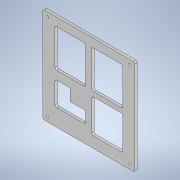
# Autodesk Inventor part: AssemblyPlate
Saved by Autodesk Inventor 2021 (Build 250183000, 183)
## iProperties
Created: 2020-11-06
Part Number: AssemblyPlate
Material: Generic
Document SubType Name: Modeling
Designer: lgnds
Density: 1 g/cm^3
Appearance: Default
Author: lgnds
Autodesk Inventor part; units mm, degrees
ref_plane "YZ Plane" through (0, 0, 0) normal (1, 0, 0) x (0, 1, 0)
ref_plane "XZ Plane" through (0, 0, 0) normal (0, 1, 0) x (-1, 0, 0)
ref_plane "XY Plane" through (0, 0, 0) normal (0, 0, 1) x (1, 0, 0)
sketch "Sketch1" plane through (0, 0, 0) normal (0, 0, 1) x (1, 0, 0)
  line L0 (-56, -58) -> (56, -58)
  line L1 (56, -58) -> (56, 58)
  line L2 (56, 58) -> (-56, 58)
  line L3 (-56, 58) -> (-56, -58)
  line L4 (-56, -58) -> (56, 58) construction
  line L5 (56, -58) -> (-56, 58) construction
  point P0 (0, 0)
  dimension "d0" = 116
  dimension "d1" = 112
  constraints: 12 end point, 2 midpoint, 2 parallel, 1 horizontal, 1 perpendicular
  measures "d0" distance between parallel lines of L0 L2
  measures "d1" distance between parallel lines of L1 L3
extrude "Extrusion1" add sketch "Sketch1" along normal blind 3
sketch "Sketch2" plane through (0, 0, 3) normal (0, 0, 1) x (1, 0, 0)
  line L0 (-78.4, 0) -> (78.4, 0) construction
  line L1 (0, 81.2) -> (0, -81.2) construction
  circle A0 centre (-50, 52.5) radius 1.5
  circle A1 centre (50, 52.5) radius 1.5
  circle A2 centre (-50, -52.5) radius 1.5
  circle A3 centre (50, -52.5) radius 1.5
  circle A4 centre (49, 0) radius 1.5
  line L2 (78.4, 0) -> (-78.4, 0) construction
  circle A5 centre (-49, 0) radius 1.5
  point P0 (0, 0)
  dimension "d4" = 3
  dimension "d5" = 100
  dimension "d6" = 105
  dimension "d44" = 3
  dimension "d45" = 98
  constraints: 6 centre point, 6 symmetric about line, 2 end point, 2 point on line, 4 other
  measures "d4" diameter of A0
  measures "d5" distance of A1.centre A0.centre
  measures "d6" distance of A3.centre A1.centre
  measures "d44" diameter of A4
  measures "d45" distance of A5.centre A4.centre
extrude "Extrusion2" cut sketch "Sketch2" against normal through all
fillet "Fillet1" radius 2 4 edges at (-56, 58, 1.5) (-56, -58, 1.5) (56, -58, 1.5) (56, 58, 1.5)
sketch "Sketch3" plane through (0, 0, 3) normal (0, 0, 1) x (1, 0, 0)
  line L0 (22.6276, -51.0248) -> (22.6276, 2.6708)
  line L1 (47.313, -24.177) -> (-2.0522, -24.177)
  line L2 (-47.3418, -22.8308) -> (2.0866, -22.8308)
  line L3 (-22.6276, -42.0332) -> (-22.6276, -3.6284)
  line L4 (2.0578, 24.9075) -> (-47.3074, 24.9075)
  line L5 (-22.6276, -5.5598) -> (-22.6276, 54.3588)
  line L6 (47.313, 24.9075) -> (-2.0522, 24.9075)
  line L7 (22.6276, -5.5598) -> (22.6276, 54.3588)
  line L8 (41.6304, -3.677) -> (3.6304, -3.677)
  line L9 (3.6304, -3.677) -> (3.6304, -44.677)
  line L10 (3.6304, -44.677) -> (41.6304, -44.677)
  line L11 (41.6304, -44.677) -> (41.6304, -3.677)
  line L12 (41.6304, -3.677) -> (3.6304, -44.677) construction
  line L13 (3.6304, -3.677) -> (41.6304, -44.677) construction
  line L14 (-4.1276, -8.3308) -> (-41.1276, -8.3308)
  line L15 (-41.1276, -8.3308) -> (-41.1276, -37.3308)
  line L16 (-41.1276, -37.3308) -> (-4.1276, -37.3308)
  line L17 (-4.1276, -37.3308) -> (-4.1276, -8.3308)
  line L18 (-4.1276, -8.3308) -> (-41.1276, -37.3308) construction
  line L19 (-41.1276, -8.3308) -> (-4.1276, -37.3308) construction
  line L20 (-4.1276, 47.9075) -> (-41.1276, 47.9075)
  line L21 (-41.1276, 47.9075) -> (-41.1276, 1.9075)
  line L22 (-41.1276, 1.9075) -> (-4.1276, 1.9075)
  line L23 (-4.1276, 1.9075) -> (-4.1276, 47.9075)
  line L24 (-4.1276, 47.9075) -> (-41.1276, 1.9075) construction
  line L25 (-41.1276, 47.9075) -> (-4.1276, 1.9075) construction
  line L26 (41.6248, 47.9075) -> (3.6304, 47.9075)
  line L27 (3.6304, 47.9075) -> (3.6304, 1.9075)
  line L28 (3.6304, 1.9075) -> (41.6248, 1.9075)
  line L29 (41.6248, 1.9075) -> (41.6248, 47.9075)
  line L30 (41.6248, 47.9075) -> (3.6304, 1.9075) construction
  line L31 (3.6304, 47.9075) -> (41.6248, 1.9075) construction
  point P0 (0, 0)
  point P1 (22.6304, -24.177)
  point P2 (-22.6276, -22.8308)
  point P3 (-22.6276, 24.9075)
  point P4 (22.6276, 24.9075)
  point P5 (-4.1276, -22.8308)
  point P6 (-22.6276, -22.8308)
  point P7 (-22.6276, -8.3308)
  dimension "d10" = 41
  dimension "d11" = 38
  dimension "d12" = 46
  dimension "d13" = 29
  dimension "d14" = 37
  dimension "d15" = 37
  constraints: 64 end point, 10 midpoint, 8 horizontal, 8 parallel, 6 point on line, 4 perpendicular, 4 vertical, 16 other
  measures "d10" distance between parallel lines of L8 L10
  measures "d11" distance between parallel lines of L9 L11
  measures "d12" distance between parallel lines of L26 L28
  measures "d13" distance between parallel lines of L14 L16
  measures "d14" distance between parallel lines of L15 L17
  measures "d15" distance between parallel lines of L21 L23
extrude "Extrusion3" cut sketch "Sketch3" against normal through all
fillet "Fillet2" radius 2 16 edges at (41.6304, -44.677, 1.5) (3.6304, -44.677, 1.5) (-4.1276, -37.3308, 1.5) (-41.1276, -37.3308, 1.5) (-41.1276, -8.3308, 1.5) (-41.1276, 1.9075, 1.5) (-41.1276, 47.9075, 1.5) (-4.1276, 47.9075, 1.5) (41.6248, 47.9075, 1.5) (3.6304, 47.9075, 1.5) (-4.1276, 1.9075, 1.5) (3.6304, 1.9075, 1.5) (41.6248, 1.9075, 1.5) (41.6304, -3.677, 1.5) (3.6304, -3.677, 1.5) (-4.1276, -8.3308, 1.5)
sketch "Sketch5" plane through (0, 0, 3) normal (0, 0, 1) x (1, 0, 0)
  circle A0 centre (-2, -3) radius 1.6
  circle A1 centre (-6, -44) radius 1.6
  circle A2 centre (40, -53) radius 1.6
  circle A3 centre (51, -42) radius 1.6
  circle A4 centre (51, -12) radius 1.6
  line L0 (56, -56) -> (56, 56) construction
  line L1 (-54, -58) -> (54, -58) construction
  line L2 (0, 81.2) -> (0, -81.2) construction
  line L3 (-78.4, 0) -> (78.4, 0) construction
  circle A5 centre (-40, -53) radius 1.6
  circle A6 centre (-51, -42) radius 1.6
  circle A7 centre (-51, -12) radius 1.6
  circle A8 centre (40, 53) radius 1.6
  circle A9 centre (51, 42) radius 1.6
  circle A10 centre (51, 12) radius 1.6
  line L4 (-54, 58) -> (54, 58) construction
  circle A11 centre (-51, 12) radius 1.6
  circle A12 centre (-51, 42) radius 1.6
  circle A13 centre (-40, 53) radius 1.6
  circle A14 centre (16, 53) radius 1.6
  circle A15 centre (-16, 53) radius 1.6
  point P0 (0, 0)
  point P1 (-56, -56)
  point P2 (-56, 56)
  dimension "d19" = 44
  dimension "d20" = 6
  dimension "d21" = 3
  dimension "d22" = 2
  dimension "d23" = 5
  dimension "d24" = 5
  dimension "d25" = 5
  dimension "d27" = 3.2
  dimension "d28" = 3.2
  dimension "d29" = 3.2
  dimension "d31" = 3.2
  dimension "d32" = 3.2
  dimension "d33" = 16
  dimension "d34" = 16
  dimension "d35" = 12
  dimension "d36" = 3.2
  dimension "d37" = 3.2
  dimension "d38" = 5
  dimension "d39" = 5
  dimension "d40" = 16
  dimension "d41" = 16
  constraints: 16 centre point, 13 symmetric about line, 2 end point, 9 other
  measures "d19" vertical distance of point (0, 0) A1.centre
  measures "d20" horizontal distance of point (0, 0) A1.centre
  measures "d21" vertical distance of point (0, 0) A0.centre
  measures "d22" horizontal distance of point (0, 0) A0.centre
  measures "d23" distance from line of L0 A4.centre
  measures "d24" distance from line of L0 A3.centre
  measures "d25" distance from line of L1 A2.centre
  measures "d27" diameter of A4
  measures "d28" diameter of A3
  measures "d29" diameter of A2
  measures "d31" diameter of A0
  measures "d32" diameter of A1
  measures "d33" distance from line of L0 A2.centre
  measures "d34" distance from line of L1 A3.centre
  measures "d35" vertical distance of point (0, 0) A4.centre
  measures "d36" diameter of A15
  measures "d37" diameter of A14
  measures "d38" distance from line of L4 A14.centre
  measures "d39" distance from line of L4 A15.centre
  measures "d40" distance from line of L2 A14.centre
  measures "d41" distance from line of L2 A15.centre
extrude "Extrusion4" cut sketch "Sketch5" against normal through all
equation "\"d44\" = d4"
equation "\"d24\" = d23"
equation "\"d25\" = d23"
equation "\"d28\" = d27"
equation "\"d29\" = d27"
equation "\"d31\" = d27"
equation "\"d32\" = d27"
equation "\"d36\" = d27"
equation "\"d37\" = d27"
equation "\"d38\" = d23"
equation "\"d39\" = d23"
equation "\"d40\" = d34"
equation "\"d41\" = d34"
body "Solid1"
